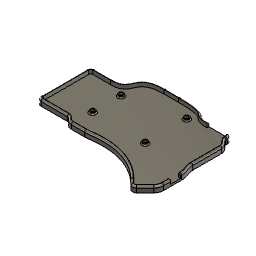
case (Autodesk Fusion 360 design; units mm, degrees)
Autodesk Fusion 360 part; units mm, degrees
note: some values were not read from the file. Chosen so that the rebuilt part matches the saved one: which bodies a step acts on. Set by a fixed rule: the direction of a hole.
sketch "holes" plane through (0, 0, 0) normal (0, 1, 0) x (1, 0, 0)
  line L0 (126.0404, -106.5892) -> (126.0404, -96.5892)
  line L1 (157.8502, -159.4086) -> (150.6767, -159.4086)
  line L2 (126.0404, -96.5892) -> (146.0404, -96.5892)
  line L3 (150.6767, -159.4086) -> (150.6767, -169.4086)
  line L4 (146.0404, -106.5892) -> (126.0404, -106.5892)
  line L5 (157.8502, -169.4086) -> (157.8502, -159.4086)
  line L6 (150.6767, -169.4086) -> (157.8502, -169.4086)
  line L7 (146.0404, -96.5892) -> (146.0404, -106.5892)
  circle A0 centre (145.3008, -163.4257) radius 0.6
  circle A1 centre (145.3008, -165.1757) radius 0.6
  circle A2 centre (54.3208, -145.8157) radius 2.5
  circle A3 centre (108.3208, -146.3157) radius 2.5
  circle A4 centre (54.3208, -116.8157) radius 2.5
  line L8 (38.8208, -162.5657) -> (47.1808, -162.5657)
  spline S0 degree 3 poles (47.1808, -162.5657) (51.7408, -162.5657) (51.7408, -167.5657) (56.3208, -167.5657) knots 1 1 1 1 2 2 2 2
  line L9 (56.3208, -167.5657) -> (69.8508, -167.5657)
  spline S1 degree 3 poles (69.8508, -167.5657) (75.9008, -167.5657) (75.8208, -166.3157) (88.3208, -166.3157) (106.4584, -166.3157) (123.8522, -173.5257) (136.6708, -186.3576) knots 3 3 3 3 4 4 4 5 5 5 5
  line L10 (136.6708, -186.3576) -> (141.4208, -191.1076)
  spline S2 degree 3 poles (141.4208, -191.1076) (142.2162, -191.8832) (143.4896, -191.8677) (144.266, -191.073) knots 6 6 6 6 7 7 7 7
  line L11 (144.266, -191.073) -> (153.0169, -182.3192)
  spline S3 degree 3 poles (153.0169, -182.3192) (154.5362, -180.8058) (155.392, -178.7508) (155.3961, -176.6064) knots 8 8 8 8 9 9 9 9
  line L12 (155.3961, -176.6064) -> (155.3961, -158.2827)
  spline S4 degree 3 poles (155.3961, -158.2827) (155.3961, -150.8157) (152.3208, -150.8157) (152.3208, -143.8257) knots 10 10 10 10 11 11 11 11
  line L13 (152.3208, -143.8257) -> (152.3208, -114.1112)
  spline S5 degree 3 poles (152.3208, -114.1112) (152.3208, -110.3657) (146.8208, -108.1957) (146.8208, -104.4757) knots 12 12 12 12 13 13 13 13
  line L14 (146.8208, -104.4757) -> (146.8208, -103.0657)
  spline S6 degree 3 poles (146.8208, -103.0657) (146.8208, -101.9611) (145.9254, -101.0657) (144.8208, -101.0657) knots 14 14 14 14 15 15 15 15
  line L15 (144.8208, -101.0657) -> (126.8208, -101.0657)
  spline S7 degree 3 poles (126.8208, -101.0657) (106.3208, -101.0657) (123.3208, -93.0657) (89.0708, -93.0657) knots 17 17 17 17 18 18 18 18
  line L16 (89.0708, -93.0657) -> (74.3308, -93.0657)
  spline S8 degree 3 poles (74.3308, -93.0657) (43.8208, -93.0657) (61.8208, -111.8157) (38.8208, -112.0657) knots 19 19 19 19 20 20 20 20
  spline S9 degree 3 poles (38.8208, -112.0657) (37.7162, -112.0657) (36.8208, -112.9611) (36.8208, -114.0657) knots 20 20 20 20 21 21 21 21
  line L17 (36.8208, -114.0657) -> (36.8208, -114.5657)
  spline S10 degree 3 poles (36.8208, -114.5657) (36.8208, -114.8418) (36.5969, -115.0657) (36.0446, -115.0657) (35.8208, -114.8418) (35.8208, -114.5657) knots 23 23 23 23 24 24 25 25 25 25
  line L18 (35.8208, -114.5657) -> (35.8208, -114.0657)
  spline S11 degree 3 poles (35.8208, -114.0657) (35.8208, -112.9611) (34.9253, -112.0657) (33.8208, -112.0657) knots 26 26 26 26 27 27 27 27
  line L19 (33.8208, -112.0657) -> (20.5708, -112.0657)
  spline S12 degree 3 poles (20.5708, -112.0657) (19.4662, -112.0657) (18.5708, -112.9611) (18.5708, -114.0657) knots 29 29 29 29 30 30 30 30
  line L20 (18.5708, -114.0657) -> (18.5708, -160.5657)
  spline S13 degree 3 poles (18.5708, -160.5657) (18.5708, -161.6703) (19.4662, -162.5657) (20.5708, -162.5657) knots 32 32 32 32 33 33 33 33
  line L21 (20.5708, -162.5657) -> (33.8208, -162.5657)
  spline S14 degree 3 poles (33.8208, -162.5657) (34.9253, -162.5657) (35.8208, -161.6703) (35.8208, -160.5657) knots 35 35 35 35 36 36 36 36
  line L22 (35.8208, -160.5657) -> (35.8208, -160.0657)
  spline S15 degree 3 poles (35.8208, -160.0657) (35.8208, -159.7895) (36.0446, -159.5657) (36.5969, -159.5657) (36.8208, -159.7895) (36.8208, -160.0657) knots 38 38 38 38 39 39 40 40 40 40
  line L23 (36.8208, -160.0657) -> (36.8208, -160.5657)
  spline S16 degree 3 poles (36.8208, -160.5657) (36.8208, -161.6703) (37.7162, -162.5657) (38.8208, -162.5657) knots 41 41 41 41 42 42 42 42
  circle A5 centre (108.3208, -103.8157) radius 2.5
extrude "Extrude7" add sketch "holes" along normal blind 4 contours A2 | A3 | A4 | A5 makes body 1 at (110.2359, 2.6667, 144.7087) makes body 2 at (56.8177, 2.6667, 116.9403) makes body 3 at (52.3279, 2.6667, 147.3252) makes body 4 at (106.328, 2.6667, 105.3252)
hole "Hole1" at (108.3208, 0, 103.8157) at (108.3208, 0, 146.3157) at (54.3208, 0, 116.8157) at (54.3208, 0, 145.8157) direction (0, 1, 0) diameter 3.3 depth 15 tip angle 180 bodies 4 1 2 3
sketch "outline" plane through (0, 0, 0) normal (0, 1, 0) x (1, 0, 0)
  line L0 (38.8208, -162.5657) -> (47.1808, -162.5657)
  spline S0 degree 3 poles (47.1808, -162.5657) (51.7408, -162.5657) (51.7408, -167.5657) (56.3208, -167.5657) knots 1 1 1 1 2 2 2 2
  line L1 (56.3208, -167.5657) -> (69.8508, -167.5657)
  spline S1 degree 3 poles (69.8508, -167.5657) (75.9008, -167.5657) (75.8208, -166.3157) (88.3208, -166.3157) (106.4584, -166.3157) (123.8522, -173.5257) (136.6708, -186.3576) knots 3 3 3 3 4 4 4 5 5 5 5
  line L2 (136.6708, -186.3576) -> (141.4208, -191.1076)
  spline S2 degree 3 poles (141.4208, -191.1076) (142.2162, -191.8832) (143.4896, -191.8677) (144.266, -191.073) knots 6 6 6 6 7 7 7 7
  line L3 (144.266, -191.073) -> (153.0169, -182.3192)
  spline S3 degree 3 poles (153.0169, -182.3192) (154.5362, -180.8058) (155.392, -178.7508) (155.3961, -176.6064) knots 8 8 8 8 9 9 9 9
  line L4 (155.3961, -176.6064) -> (155.3961, -158.2827)
  spline S4 degree 3 poles (155.3961, -158.2827) (155.3961, -150.8157) (152.3208, -150.8157) (152.3208, -143.8257) knots 10 10 10 10 11 11 11 11
  line L5 (152.3208, -143.8257) -> (152.3208, -114.1112)
  spline S5 degree 3 poles (152.3208, -114.1112) (152.3208, -110.3657) (146.8208, -108.1957) (146.8208, -104.4757) knots 12 12 12 12 13 13 13 13
  line L6 (146.8208, -104.4757) -> (146.8208, -103.0657)
  spline S6 degree 3 poles (146.8208, -103.0657) (146.8208, -101.9611) (145.9254, -101.0657) (144.8208, -101.0657) knots 14 14 14 14 15 15 15 15
  line L7 (144.8208, -101.0657) -> (126.8208, -101.0657)
  spline S7 degree 3 poles (126.8208, -101.0657) (106.3208, -101.0657) (123.3208, -93.0657) (89.0708, -93.0657) knots 17 17 17 17 18 18 18 18
  line L8 (89.0708, -93.0657) -> (74.3308, -93.0657)
  spline S8 degree 3 poles (74.3308, -93.0657) (43.8208, -93.0657) (61.8208, -111.8157) (38.8208, -112.0657) knots 19 19 19 19 20 20 20 20
  spline S9 degree 3 poles (38.8208, -112.0657) (37.7162, -112.0657) (36.8208, -112.9611) (36.8208, -114.0657) knots 20 20 20 20 21 21 21 21
  line L9 (36.8208, -114.0657) -> (36.8208, -114.5657)
  spline S10 degree 3 poles (36.8208, -114.5657) (36.8208, -114.8418) (36.5969, -115.0657) (36.0446, -115.0657) (35.8208, -114.8418) (35.8208, -114.5657) knots 23 23 23 23 24 24 25 25 25 25
  line L10 (35.8208, -114.5657) -> (35.8208, -114.0657)
  spline S11 degree 3 poles (35.8208, -114.0657) (35.8208, -112.9611) (34.9253, -112.0657) (33.8208, -112.0657) knots 26 26 26 26 27 27 27 27
  line L11 (33.8208, -112.0657) -> (20.5708, -112.0657)
  spline S12 degree 3 poles (20.5708, -112.0657) (19.4662, -112.0657) (18.5708, -112.9611) (18.5708, -114.0657) knots 29 29 29 29 30 30 30 30
  line L12 (18.5708, -114.0657) -> (18.5708, -160.5657)
  spline S13 degree 3 poles (18.5708, -160.5657) (18.5708, -161.6703) (19.4662, -162.5657) (20.5708, -162.5657) knots 32 32 32 32 33 33 33 33
  line L13 (20.5708, -162.5657) -> (33.8208, -162.5657)
  spline S14 degree 3 poles (33.8208, -162.5657) (34.9253, -162.5657) (35.8208, -161.6703) (35.8208, -160.5657) knots 35 35 35 35 36 36 36 36
  line L14 (35.8208, -160.5657) -> (35.8208, -160.0657)
  spline S15 degree 3 poles (35.8208, -160.0657) (35.8208, -159.7895) (36.0446, -159.5657) (36.5969, -159.5657) (36.8208, -159.7895) (36.8208, -160.0657) knots 38 38 38 38 39 39 40 40 40 40
  line L15 (36.8208, -160.0657) -> (36.8208, -160.5657)
  spline S16 degree 3 poles (36.8208, -160.5657) (36.8208, -161.6703) (37.7162, -162.5657) (38.8208, -162.5657) knots 41 41 41 41 42 42 42 42
  line L16 (33.2075, -112.0657) -> (38.8208, -112.0657)
  line L17 (33.8208, -162.5657) -> (38.8208, -162.5657)
  line L18 (33.8208, -164.5657) -> (38.8208, -164.5657)
  line L19 (38.8208, -164.5657) -> (47.1808, -164.5657)
  spline S17 degree 3 poles (47.1808, -164.5657) (47.9255, -164.5657) (48.3166, -164.719) (48.739, -164.9853) (49.2686, -165.3193) (49.824, -165.9402) (50.5638, -166.7381) (51.2305, -167.4572) (52.0736, -168.3226) (53.316, -168.9141) (54.1698, -169.3205) (55.1944, -169.5657) (56.3208, -169.5657) knots 1 1 1 1 1.240396 1.240396 1.240396 1.541779 1.541779 1.541779 1.813372 1.813372 1.813372 2 2 2 2
  line L20 (56.3208, -169.5657) -> (69.8508, -169.5657)
  spline S18 degree 3 poles (69.8508, -169.5657) (72.5889, -169.5657) (74.2411, -169.3087) (76.0649, -169.0453) (78.0115, -168.7641) (80.2474, -168.4606) (84.8201, -168.3537) (85.8608, -168.3294) (87.0205, -168.3157) (88.3208, -168.3157) (105.9284, -168.3157) (122.8118, -175.3141) (135.2558, -187.771) (135.256, -187.7712) (135.2561, -187.7713) (135.2562, -187.7714) knots 3 3 3 3 3.432865 3.432865 3.432865 3.894855 3.894855 3.894855 4 4 4 5 5 5 5.000009 5.000009 5.000009 5.000009
  line L21 (135.2562, -187.7714) -> (140.0155, -192.5307)
  spline S19 degree 3 poles (140.0155, -192.5307) (140.0185, -192.5336) (140.0215, -192.5365) (140.0245, -192.5395) (141.0715, -193.5605) (142.5633, -193.9014) (143.8933, -193.5352) (144.5519, -193.3538) (145.1797, -192.9963) (145.6872, -192.4802) knots 5.996226 5.996226 5.996226 5.996226 6 6 6 6.667423 6.667423 6.667423 6.99795 6.99795 6.99795 6.99795
  line L22 (145.6872, -192.4802) -> (154.4284, -183.7361)
  spline S20 degree 3 poles (154.4284, -183.7361) (156.3229, -181.8489) (157.391, -179.2844) (157.3961, -176.6103) knots 8 8 8 8 9 9 9 9
  line L23 (157.3961, -176.6103) -> (157.3961, -158.2827)
  spline S21 degree 3 poles (157.3961, -158.2827) (157.3961, -155.3354) (156.92, -153.2828) (156.3341, -151.6724) (155.8477, -150.3354) (155.3439, -149.351) (154.9852, -148.3007) (154.6009, -147.1753) (154.3208, -145.9201) (154.3208, -143.8257) knots 10 10 10 10 10.367667 10.367667 10.367667 10.672919 10.672919 10.672919 11 11 11 11
  line L24 (154.3208, -143.8257) -> (154.3208, -114.1112)
  spline S22 degree 3 poles (154.3208, -114.1112) (154.3208, -112.8332) (153.8866, -111.695) (153.3323, -110.7686) (152.4936, -109.3669) (151.3985, -108.3268) (150.5294, -107.3754) (149.8258, -106.6052) (149.2818, -105.9073) (149.0302, -105.3526) (148.8814, -105.0244) (148.8208, -104.7596) (148.8208, -104.4757) knots 12 12 12 12 12.22408 12.22408 12.22408 12.563116 12.563116 12.563116 12.83762 12.83762 12.83762 13 13 13 13
  line L25 (148.8208, -104.4757) -> (148.8208, -103.0657)
  spline S23 degree 3 poles (148.8208, -103.0657) (148.8208, -101.6086) (148.0267, -100.3074) (146.8409, -99.6129) (146.2481, -99.2657) (145.5492, -99.0657) (144.8208, -99.0657) knots 14 14 14 14 14.666701 14.666701 14.666701 15 15 15 15
  line L26 (144.8208, -99.0657) -> (126.8208, -99.0657)
  spline S24 degree 3 poles (126.8208, -99.0657) (122.7932, -99.0657) (120.3545, -98.7388) (118.8189, -98.2989) (117.3999, -97.8923) (116.7415, -97.4486) (115.9604, -96.8255) (115.2716, -96.276) (114.4891, -95.5233) (113.3053, -94.7611) (111.9186, -93.8683) (110.0373, -93.0363) (107.196, -92.4121) (103.4227, -91.5832) (97.9013, -91.0657) (89.0708, -91.0657) knots 17 17 17 17 17.201582 17.201582 17.201582 17.38785 17.38785 17.38785 17.552108 17.552108 17.552108 17.744498 17.744498 17.744498 18 18 18 18
  line L27 (89.0708, -91.0657) -> (74.3308, -91.0657)
  spline S25 degree 3 poles (74.3308, -91.0657) (67.5023, -91.0657) (62.8681, -91.9661) (59.5165, -93.5424) (56.6795, -94.8767) (54.8159, -96.7408) (53.5601, -98.6489) (52.2214, -100.6831) (51.5061, -102.7112) (50.6894, -104.3575) (50.0131, -105.7206) (49.3103, -106.8089) (48.2216, -107.693) (47.1199, -108.5876) (45.5591, -109.3383) (42.9359, -109.7524) (41.7733, -109.936) (40.4084, -110.0479) (38.8098, -110.0657) knots 19 19 19 19 19.217959 19.217959 19.217959 19.402457 19.402457 19.402457 19.599145 19.599145 19.599145 19.761998 19.761998 19.761998 19.926797 19.926797 19.926797 19.999837 19.999837 19.999837 19.999837
  line L28 (33.2075, -110.0657) -> (38.8098, -110.0657)
  line L29 (33.8208, -110.0657) -> (20.5708, -110.0657)
  spline S26 degree 3 poles (20.5708, -110.0657) (19.1137, -110.0657) (17.8126, -110.8598) (17.118, -112.0455) (16.7708, -112.6383) (16.5708, -113.3373) (16.5708, -114.0657) knots 29 29 29 29 29.666696 29.666696 29.666696 30 30 30 30
  line L30 (16.5708, -114.0657) -> (16.5708, -160.5657)
  spline S27 degree 3 poles (16.5708, -160.5657) (16.5708, -162.0227) (17.3649, -163.3239) (18.5506, -164.0184) (19.1434, -164.3656) (19.8424, -164.5657) (20.5708, -164.5657) knots 32 32 32 32 32.666699 32.666699 32.666699 33 33 33 33
  line L31 (20.5708, -164.5657) -> (33.8208, -164.5657)
  dimension "d33" = -2
  dimension "d34" = 2
  constraint coincident L11 L16.start
  constraint parallel L11 L16
extrude "Extrude8" add sketch "outline" along normal blind 6 separate body makes body 5
extrude "Extrude9" add sketch "outline" along normal blind 2 contours L0 S0 L1 S1 L2 S2 L3 S3 L4 S4 L5 S5 L6 S6 L7 S7 L8 S8 S9 L9 S10 L10 S11 L11 S12 L12 S13 L13 S14 L14 S15 L15 S16 L16 | S14 L14 S15 L15 S16 L17 | S9 L9 S10 L10 S11 L16 bodies 4 1 2 3 5
extrude "Extrude11" cut sketch "holes" along normal blind 20 from surface at 2 contours L0 L4 L7 S6 L15 S7 | L0 L2 L7 S6 L15 S7 | L1 L3 L6 L12 | L1 L5 L6 L12 bodies 4
fillet "Fillet2" radius 1.8 22 edges at (29.6903, 6, 110.0657) (17.7457, 6, 111.2358) (16.5708, 6, 137.3157) (17.7409, 6, 163.3907) (33.8758, 6, 164.5657) (50.2663, 6, 166.4168) (63.0858, 6, 169.5657) (88.321, 6, 168.3157) (137.6358, 6, 190.151) (114.2019, 6, 95.3872) (81.7008, 6, 91.0657) (51.9411, 6, 101.6226) (157.3961, 6, 158.8456) (155.705, 6, 150.0982) (154.3208, 6, 128.9684) (151.0352, 6, 107.9177) (148.8208, 6, 103.7707) (148.037, 6, 100.6909) (157.3961, 6, 173.0094) (156.6208, 6, 180.4683) (150.0578, 6, 188.1082) (142.8534, 6, 193.6778) on bodies 4 5
chamfer "Chamfer2" distance 1 angle 45 4 edges at (51.99, 2, 117.7197) (51.99, 2, 146.7197) (105.99, 2, 147.2197) (105.99, 2, 104.7197) on bodies 4
named bodies: "case"
